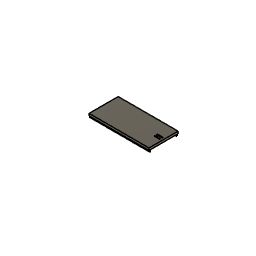
StructureTop (Autodesk Fusion 360 design; units mm, degrees)
Autodesk Fusion 360 part; units mm, degrees
sketch "Sketch1" plane through (0, 0, 38.5922) normal (0, 0, 1) x (-1, 0, 0)
  line L0 (-33.763, -0.9939) -> (33.5, -0.9939)
  line L1 (33.5, -0.9939) -> (33.5, 1.0061)
  line L2 (33.5, 1.0061) -> (-33.763, 1.0061)
  line L3 (-33.763, 1.0061) -> (-33.763, -0.9939)
  line L4 (-33.763, 1.0061) -> (33.497, 1.0061)
  line L5 (33.497, 1.0061) -> (33.497, -16.9939)
  line L6 (33.497, -16.9939) -> (-33.763, -16.9939)
  line L7 (-33.763, -16.9939) -> (-33.763, 1.0061)
  line L8 (-33.763, -2.0276) -> (33.5, -2.0276)
  line L9 (33.5, -2.0276) -> (33.5, -0.9939)
  line L10 (33.5, -0.9939) -> (-33.763, -0.9939)
  line L11 (-33.763, -0.9939) -> (-33.763, -2.0276)
  line L12 (33.499, -14) -> (-33.763, -14)
  line L13 (-33.763, -14) -> (-33.763, -15.0005)
  line L14 (-33.763, -15.0005) -> (33.499, -15.0005)
  line L15 (33.499, -15.0005) -> (33.499, -14)
  dimension "d80" = 18
  constraint horizontal L4
  constraint vertical L5
  constraint horizontal L6
  constraint vertical L7
  constraint coincident L2.end L3.start
  constraint horizontal L8
  constraint vertical L9
  constraint horizontal L10
  constraint vertical L11
  constraint coincident L0.end L1.start
  constraint coincident L7 L8.start
  constraint horizontal L12
  constraint vertical L13
  constraint horizontal L14
  constraint vertical L15
  constraint coincident L7 L13.end
  measures "d80" distance of L2.end L6.end
extrude "Extrude1" add sketch "Sketch1" along normal blind 2.5 contours L0 L2 L3 L4 L5 L7 L10 | L0 L5 L7 L8 L10 L11 | L5 L7 L8 L12 | L5 L7 L12 L13 L14 | L5 L6 L7 L14 picked at (-11.343, 0.3394) picked at (11.077, -1.683) picked at (-11.343, -10.0092) picked at (-11.343, -14.3335) picked at (-11.343, -15.665)
sketch "Sketch4" plane through (0, 0, 41.0922) normal (0, 0, 1) x (-1, 0, 0)
  line L0 (-33.763, 1.0061) -> (-33.763, -16.9939)
  line L1 (-33.763, -16.9939) -> (33.497, -16.9939)
  line L2 (33.497, -16.9939) -> (33.497, 1.0061)
  line L3 (33.497, 1.0061) -> (-33.763, 1.0061)
  line L4 (-31.263, -18) -> (-31.263, 4.3676) construction
  line L5 (-31.263, -7.0873) -> (-25.263, -7.0873)
  line L6 (-25.263, -7.0873) -> (-25.263, -6.0873)
  line L7 (-25.263, -6.0873) -> (-31.263, -6.0873)
  line L8 (-31.263, -6.0873) -> (-31.263, -7.0873)
  line L9 (-31.263, -9.8361) -> (-25.263, -9.8361)
  line L10 (-25.263, -9.8361) -> (-25.263, -8.8361)
  line L11 (-25.263, -8.8361) -> (-31.263, -8.8361)
  line L12 (-31.263, -8.8361) -> (-31.263, -9.8361)
  dimension "d93" = 2.5
  dimension "d94" = 6
  dimension "d95" = 1
  dimension "d96" = 6
  dimension "d97" = 1
  constraint perpendicular L3 L4
  constraint horizontal L5
  constraint vertical L6
  constraint horizontal L7
  constraint vertical L8
  constraint coincident L4 L5.start
  constraint horizontal L9
  constraint vertical L10
  constraint horizontal L11
  constraint vertical L12
  constraint coincident L4 L9.start
  measures "d93" distance of L0 L4
  measures "d94" distance of L5.start L5.end
  measures "d95" distance of L5.start L7.end
  measures "d96" distance of L9.start L9.end
  measures "d97" distance of L9.start L11.end
extrude "Extrude5" cut sketch "Sketch4" against normal blind 2.5 contours L5 L6 L7 L8 | L9 L10 L11 L12 picked at (-29.263, -6.7539) picked at (-29.263, -9.5028)
move_face "OffsetFaces3" offset 7.35 2 faces at (-11.077, 16.9939, 40.2589) (-11.077, -1.0061, 39.4255)
sketch "Sketch5" plane through (0, 0, 38.5922) normal (0, 0, -1) x (1, 0, 0)
  line L0 (31.263, -7.0873) -> (25.263, -7.0873)
  line L1 (25.263, -7.0873) -> (25.263, -6.0873)
  line L2 (25.263, -6.0873) -> (31.263, -6.0873)
  line L3 (31.263, -6.0873) -> (31.263, -7.0873)
  line L4 (31.263, -9.8361) -> (25.263, -9.8361)
  line L5 (25.263, -9.8361) -> (25.263, -8.8361)
  line L6 (25.263, -8.8361) -> (31.263, -8.8361)
  line L7 (31.263, -8.8361) -> (31.263, -9.8361)
  line L8 (33.763, -24.3439) -> (33.763, 8.3561)
  line L9 (33.763, 8.3561) -> (-33.497, 8.3561)
  line L10 (-33.497, 8.3561) -> (-33.497, -24.3439)
  line L11 (-33.497, -24.3439) -> (33.763, -24.3439)
  line L12 (33.763, 7.4811) -> (-33.497, 7.4811)
  line L13 (-33.497, 7.4811) -> (-33.497, 6.7311)
  line L14 (-33.497, 6.7311) -> (33.763, 6.7311)
  line L15 (33.763, 6.7311) -> (33.763, 7.4811)
  line L16 (33.763, -22.7189) -> (-33.497, -22.7189)
  line L17 (-33.497, -22.7189) -> (-33.497, -23.4689)
  line L18 (-33.497, -23.4689) -> (33.763, -23.4689)
  line L19 (33.763, -23.4689) -> (33.763, -22.7189)
  dimension "d249" = 0.75
  dimension "d250" = 0.875
  dimension "d251" = 0.75
  dimension "d252" = 0.875
  constraint horizontal L12
  constraint vertical L13
  constraint horizontal L14
  constraint vertical L15
  constraint coincident L10 L13.end
  constraint coincident L8 L12.start
  constraint horizontal L16
  constraint vertical L17
  constraint horizontal L18
  constraint vertical L19
  constraint coincident L10 L17.end
  constraint coincident L8 L16.start
  measures "d249" distance of L12.start L14.end
  measures "d250" distance of L9 L12
  measures "d251" distance of L16.start L18.end
  measures "d252" distance of L11 L18
extrude "Extrude7" add sketch "Sketch5" along normal blind 1.9 contours L8 L10 L16 L17 L18 L19 | L8 L10 L12 L13 L14 L15 picked at (-11.077, -23.2189) picked at (-11.077, 6.9811)
